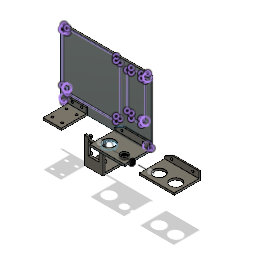
eye control mount (Autodesk Fusion 360 design; units mm, degrees)
Autodesk Fusion 360 part; units mm, degrees
sketch "Sketch1" plane through (0, 0, 0) normal (0, 0, 1) x (1, 0, 0)
  line L0 (-48.1387, 52.6701) -> (69.8353, 52.6701)
  line L1 (74.8353, 47.6701) -> (74.8353, -36.3099)
  line L2 (69.8353, -41.3099) -> (-48.1387, -41.3099)
  line L3 (-53.1387, -36.3099) -> (-53.1387, 47.6701)
  circle A0 centre (-46.9562, 49.6701) radius 1.5
  circle A1 centre (28.0438, 49.6701) radius 1.5
  circle A2 centre (-46.9562, -25.3299) radius 1.5
  circle A3 centre (28.0438, -25.3299) radius 1.5
  circle A4 centre (44.5655, 44.7298) radius 1
  circle A5 centre (63.5655, 44.7298) radius 1
  circle A6 centre (44.5655, -10.2702) radius 1
  circle A7 centre (63.5655, -10.2702) radius 1
  circle A8 centre (35.5562, -33.2226) radius 1.5
  circle A9 centre (65.5562, -33.2226) radius 1.5
  line L4 (25.4808, 51.0503) -> (25.4808, -28.2231)
  line L5 (-43.7955, -28.2231) -> (-43.7955, 51.0503)
  line L6 (41.0452, 42.402) -> (66.5755, 42.402)
  line L7 (66.5755, 42.402) -> (66.5755, -7.4237)
  line L8 (66.5755, -7.4237) -> (41.0452, -7.4237)
  line L9 (41.0452, -7.4237) -> (41.0452, 42.402)
  arc A10 (-48.1387, 52.6701) -> (-53.1387, 47.6701) centre (-48.1387, 47.6701) ccw
  arc A11 (74.8353, 47.6701) -> (69.8353, 52.6701) centre (69.8353, 47.6701) ccw
  arc A12 (69.8353, -41.3099) -> (74.8353, -36.3099) centre (69.8353, -36.3099) ccw
  arc A13 (-53.1387, -36.3099) -> (-48.1387, -41.3099) centre (-48.1387, -36.3099) ccw
  line L10 (46.8017, 47.9311) -> (61.294, 47.9311)
  line L11 (61.294, 47.9311) -> (61.294, -14.0499)
  line L12 (61.294, -14.0499) -> (46.8017, -14.0499)
  line L13 (46.8017, -14.0499) -> (46.8017, 47.9311)
  line L14 (-43.7955, -28.2231) -> (25.4808, -28.2231)
  line L15 (-43.7955, 51.0503) -> (25.4808, 51.0503)
  line L16 (-50.5532, 46.1259) -> (31.0875, 46.1259)
  line L17 (31.0875, 46.1259) -> (31.0875, -21.9998)
  line L18 (31.0875, -21.9998) -> (-50.5532, -21.9998)
  line L19 (-50.5532, -21.9998) -> (-50.5532, 46.1259)
  dimension "d1" = 3
  dimension "d4" = 75
  dimension "d5" = -75
  dimension "d6" = 2
  dimension "d9" = 19
  dimension "d10" = -55
  dimension "d11" = 3
  dimension "d14" = 30
  dimension "d15" = 0
  dimension "d30" = 5
  dimension "d31" = 5
  dimension "d59" = 8.0873
  dimension "d60" = 127.974
  dimension "d61" = 3
  dimension "d62" = 93.98
  dimension "d63" = 69.2762
  dimension "d65" = 75
  dimension "d66" = 75
  constraint horizontal L0
  constraint vertical L1
  constraint horizontal L2
  constraint vertical L3
  constraint vertical L4
  constraint vertical L5
  constraint horizontal L6
  constraint vertical L7
  constraint horizontal L8
  constraint vertical L9
  constraint tangent L0 A10
  constraint tangent L3 A10
  constraint tangent L0 A11
  constraint tangent L1 A11
  constraint tangent L1 A12
  constraint tangent L2 A12
  constraint equal A11 A12
  constraint tangent L2 A13
  constraint tangent L3 A13
  constraint equal A11 A13
  constraint horizontal L10
  constraint vertical L11
  constraint horizontal L12
  constraint vertical L13
  constraint horizontal L14
  constraint horizontal L15
  constraint horizontal L16
  constraint vertical L17
  constraint horizontal L18
  constraint vertical L19
  constraint coincident L5.end L15.start
  constraint coincident L4.start L15.end
  constraint coincident L5.start L14.start
  constraint coincident L4.end L14.end
  measures "d1" diameter of A0
  measures "d6" diameter of A4
  measures "d11" diameter of A8
  measures "d30" radius of A10
  measures "d31" radius of A11
  measures "d59" distance of L2 A8.centre
  measures "d60" distance of L1 L3
  measures "d61" distance of L0 A0.centre
  measures "d62" distance of L0 L2
  measures "d63" distance of L5.end L4.start
  measures "d65" distance of A0.centre A1.centre
  measures "d66" distance of A0.centre A2.centre
extrude "Extrude1" add sketch "Sketch1" along normal blind 2 makes body 1
sketch "Sketch2" plane through (0, 0, 0) normal (0, 0, -1) x (-1, 0, 0)
  circle A0 centre (46.9562, 49.6701) radius 1.5
  circle A1 centre (-28.0438, 49.6701) radius 1.5
  circle A2 centre (-63.5655, 44.7298) radius 1
  circle A3 centre (-28.0438, -25.3299) radius 1.5
  circle A4 centre (-44.5655, 44.7298) radius 1
  circle A5 centre (-65.5562, -33.2226) radius 1.5
  line L0 (43.7955, 51.0503) -> (43.7955, 46.1259)
  circle A6 centre (-44.5655, -10.2702) radius 1
  line L1 (-61.294, -7.4237) -> (-66.5755, -7.4237)
  line L2 (-66.5755, -7.4237) -> (-66.5755, 42.402)
  line L3 (-66.5755, 42.402) -> (-61.294, 42.402)
  line L4 (-41.0452, 42.402) -> (-41.0452, -7.4237)
  circle A7 centre (-63.5655, -10.2702) radius 1
  circle A8 centre (46.9562, -25.3299) radius 1.5
  circle A9 centre (-35.5562, -33.2226) radius 1.5
  line L5 (-69.8353, -41.3099) -> (48.1387, -41.3099)
  line L6 (53.1387, -36.3099) -> (53.1387, 47.6701)
  line L7 (48.1387, 52.6701) -> (-69.8353, 52.6701)
  line L8 (-74.8353, 47.6701) -> (-74.8353, -36.3099)
  arc A10 (53.1387, 47.6701) -> (48.1387, 52.6701) centre (48.1387, 47.6701) ccw
  arc A11 (-69.8353, 52.6701) -> (-74.8353, 47.6701) centre (-69.8353, 47.6701) ccw
  arc A12 (-74.8353, -36.3099) -> (-69.8353, -41.3099) centre (-69.8353, -36.3099) ccw
  arc A13 (48.1387, -41.3099) -> (53.1387, -36.3099) centre (48.1387, -36.3099) ccw
  line L9 (-61.294, 42.402) -> (-61.294, 47.9311)
  line L10 (-46.8017, 47.9311) -> (-46.8017, 42.402)
  line L11 (-46.8017, 42.402) -> (-41.0452, 42.402)
  line L12 (-25.4808, -21.9998) -> (-31.0875, -21.9998)
  line L13 (-31.0875, -21.9998) -> (-31.0875, 46.1259)
  line L14 (-31.0875, 46.1259) -> (-25.4808, 46.1259)
  line L15 (43.7955, -28.2231) -> (-25.4808, -28.2231)
  line L16 (-25.4808, -28.2231) -> (-25.4808, -21.9998)
  line L17 (-25.4808, 46.1259) -> (-25.4808, 51.0503)
  line L18 (-25.4808, 51.0503) -> (43.7955, 51.0503)
  line L19 (43.7955, 46.1259) -> (50.5532, 46.1259)
  line L20 (50.5532, 46.1259) -> (50.5532, -21.9998)
  line L21 (50.5532, -21.9998) -> (43.7955, -21.9998)
  line L22 (43.7955, -21.9998) -> (43.7955, -28.2231)
  line L23 (-41.0452, -7.4237) -> (-46.8017, -7.4237)
  line L24 (-46.8017, -14.0499) -> (-61.294, -14.0499)
  line L25 (-61.294, -14.0499) -> (-61.294, -7.4237)
  line L26 (-61.294, 47.9311) -> (-46.8017, 47.9311)
  line L27 (-46.8017, -7.4237) -> (-46.8017, -14.0499)
extrude "Extrude2" add sketch "Sketch2" along normal blind 0.6 contours L0 L12 L13 L14 L15 L16 L17 L18 L19 L20 L21 L22 | L1 L2 L3 L4 L9 L10 L11 L23 L24 L25 L26 L27 | L5 L6 L7 L8 A10 A11 A12 A13 bodies 1
sketch "Sketch1 (2)" plane through (0, 0, 2) normal (0, 0, 1) x (1, 0, 0) in component "switch mount"
  circle A0 centre (65.5562, -33.2226) radius 1.5
  circle A1 centre (63.5655, 44.7298) radius 1
  circle A2 centre (-46.9562, 49.6701) radius 1.5
  circle A3 centre (28.0438, 49.6701) radius 1.5
  circle A4 centre (-46.9562, -25.3299) radius 1.5
  circle A5 centre (44.5655, 44.7298) radius 1
  circle A6 centre (44.5655, -10.2702) radius 1
  circle A7 centre (63.5655, -10.2702) radius 1
  circle A8 centre (35.5562, -33.2226) radius 1.5
  circle A9 centre (28.0438, -25.3299) radius 1.5
  line L0 (-48.1387, -41.3099) -> (69.8353, -41.3099)
  line L1 (74.8353, -36.3099) -> (74.8353, 47.6701)
  line L2 (69.8353, 52.6701) -> (-48.1387, 52.6701)
  line L3 (-53.1387, 47.6701) -> (-53.1387, -36.3099)
  line L4 (36.9358, -28.4317) -> (74.2813, -28.4317)
  line L5 (74.2813, -28.4317) -> (74.2813, -40.7433)
  line L6 (74.2813, -40.7433) -> (25.2813, -40.7433)
  line L7 (25.2813, -40.7433) -> (25.2813, -34.7351)
  line L8 (-43.7955, -28.2231) -> (-43.7955, -21.9998)
  line L9 (66.5755, -7.4237) -> (61.294, -7.4237)
  line L10 (41.0452, -7.4237) -> (41.0452, 42.402)
  line L11 (41.0452, 42.402) -> (46.8017, 42.402)
  line L12 (66.5755, 42.402) -> (66.5755, -7.4237)
  arc A10 (-48.1387, 52.6701) -> (-53.1387, 47.6701) centre (-48.1387, 47.6701) ccw
  arc A11 (-53.1387, -36.3099) -> (-48.1387, -41.3099) centre (-48.1387, -36.3099) ccw
  arc A12 (69.8353, -41.3099) -> (74.8353, -36.3099) centre (69.8353, -36.3099) ccw
  arc A13 (74.8353, 47.6701) -> (69.8353, 52.6701) centre (69.8353, 47.6701) ccw
  line L13 (46.8017, -14.0499) -> (46.8017, -7.4237)
  line L14 (61.294, 47.9311) -> (61.294, 42.402)
  line L15 (61.294, 42.402) -> (66.5755, 42.402)
  line L16 (-50.5532, 46.1259) -> (-43.7955, 46.1259)
  line L17 (31.0875, 46.1259) -> (31.0875, -21.9998)
  line L18 (-43.7955, -21.9998) -> (-50.5532, -21.9998)
  line L19 (25.4808, -28.2231) -> (-43.7955, -28.2231)
  line L20 (-50.5532, -21.9998) -> (-50.5532, 46.1259)
  line L21 (-43.7955, 46.1259) -> (-43.7955, 51.0503)
  line L22 (-43.7955, 51.0503) -> (25.4808, 51.0503)
  line L23 (25.4808, 51.0503) -> (25.4808, 46.1259)
  line L24 (25.4808, -21.9998) -> (25.4808, -28.2231)
  line L25 (46.8017, -7.4237) -> (41.0452, -7.4237)
  line L26 (61.294, -14.0499) -> (46.8017, -14.0499)
  line L27 (46.8017, 47.9311) -> (61.294, 47.9311)
  line L28 (61.294, -7.4237) -> (61.294, -14.0499)
  line L29 (36.9358, -28.4317) -> (25.2813, -34.7351)
  line L30 (46.8017, 42.402) -> (46.8017, 47.9311)
  line L31 (25.4808, 46.1259) -> (31.0875, 46.1259)
  line L32 (31.0875, -21.9998) -> (25.4808, -21.9998)
  dimension "d55" = 49
  dimension "d56" = 12.3116
  dimension "d57" = 10.2749
  dimension "d58" = 4.7908
  constraint horizontal L4
  constraint vertical L5
  constraint horizontal L6
  constraint vertical L7
  measures "d55" distance of L5 L7
  measures "d56" distance of L4 L6
  measures "d57" distance of A8.centre L7
  measures "d58" distance of A8.centre L4
extrude "Extrude1'" add sketch "Sketch1 (2)" along normal blind 2 separate body contours L5 L6 A12 | L4 L5 L6 L7 A12 L29 makes body 2 in component "switch mount"
sketch "Sketch2 (2)" plane through (0, 0, 4) normal (0, 0, 1) x (1, 0, 0) in component "switch mount"
  circle A0 centre (65.5562, -33.2226) radius 1.5
  circle A1 centre (35.5562, -33.2226) radius 1.5
  line L0 (25.2813, -40.7433) -> (74.2813, -40.7433)
  line L1 (74.2813, -40.7433) -> (74.2813, -28.4317)
  line L2 (74.2813, -28.4317) -> (36.9358, -28.4317)
  line L3 (25.2813, -34.7351) -> (25.2813, -40.7433)
  line L4 (25.2813, -37.7433) -> (74.2813, -37.7433)
  line L5 (36.9358, -28.4317) -> (25.2813, -34.7351)
  dimension "d20" = 3
  constraint coincident L3 L4.start
  constraint coincident L1 L4.end
  constraint perpendicular L1 L4
  measures "d20" distance of L0 L4
extrude "Extrude2'" add sketch "Sketch2 (2)" along normal blind 35 contours L0 L1 L3 L4 bodies 2 in component "switch mount"
sketch "Sketch3" plane through (0, -40.7433, 0) normal (0, -1, 0) x (1, 0, 0) in component "switch mount"
  line L0 (25.2813, 2) -> (74.2813, 2)
  line L1 (74.2813, 2) -> (74.2813, 39)
  line L2 (74.2813, 39) -> (25.2813, 39)
  line L3 (25.2813, 39) -> (25.2813, 2)
  circle A0 centre (61.9113, 27) radius 5
  circle A1 centre (37.2813, 23.82) radius 8
  line L4 (27.2813, 27) -> (98.2678, 27) construction
  line L5 (74.2813, 29) -> (72.2813, 29)
  line L6 (72.2813, 29) -> (72.2813, 25)
  line L7 (72.2813, 25) -> (74.2813, 25)
  line L8 (74.2813, 25) -> (74.2813, 29)
  dimension "d23" = 10
  dimension "d50" = 16
  dimension "d53" = 12
  dimension "d81" = 12
  dimension "d82" = 12.37
  dimension "d83" = 2
  dimension "d84" = 2
  dimension "d85" = 2
  constraint coincident A0.centre L4
  constraint horizontal L5
  constraint vertical L6
  constraint horizontal L7
  constraint vertical L8
  constraint coincident L1 L5.start
  measures "d23" diameter of A0
  measures "d50" diameter of A1
  measures "d53" distance of L2 A0.centre
  measures "d81" distance of L3 A1.centre
  measures "d82" distance of L1 A0.centre
  measures "d83" distance of L6 L8
  measures "d84" distance of L4 L5
  measures "d85" distance of L4 L7
extrude "Extrude1''" add 1 faces at (74.2813, -39.7433, 15) along direction (1, 0, 0) blind 26 separate body on bodies 2 makes body 3 in component "eye power mount"
sketch "Sketch2 (3)" plane through (0, -40.7433, 0) normal (0, -1, 0) x (1, 0, 0) in component "eye power mount"
  line L0 (74.2813, 39) -> (74.2813, 2)
  line L1 (74.2813, 2) -> (100.2813, 2)
  line L2 (100.2813, 2) -> (100.2813, 39)
  line L3 (100.2813, 39) -> (74.2813, 39)
  circle A0 centre (80.2639, 31.6259) radius 1.5
  circle A1 centre (94.2639, 31.6259) radius 1.5
  circle A2 centre (80.2639, 11.6259) radius 1.5
  circle A3 centre (94.2639, 11.6259) radius 1.5
  dimension "d34" = 3
  dimension "d37" = 14
  dimension "d38" = -20
  dimension "d69" = 7.3741
  dimension "d70" = 5.9827
  measures "d34" diameter of A0
  measures "d69" distance of L3 A0.centre
  measures "d70" distance of L0 A0.centre
extrude "Extrude2''" cut sketch "Sketch2 (3)" against normal up to surface (3 mm away) contours A0 | A1 | A2 | A3 bodies 3 in component "eye power mount"
sketch "Sketch3 (2)" plane through (0, 0, 4) normal (0, 0, 1) x (1, 0, 0) in component "eye power mount"
  line L0 (74.2813, -28.4317) -> (74.2813, -37.7433)
  line L1 (74.2813, -37.7433) -> (100.2813, -37.7433)
  line L2 (100.2813, -37.7433) -> (100.2813, -28.4317)
  line L3 (100.2813, -28.4317) -> (74.2813, -28.4317)
  circle A0 centre (93.6757, -32.8867) radius 1.5
  circle A1 centre (80.6757, -32.8867) radius 1.5
  dimension "d41" = 3
  dimension "d44" = -13
  dimension "d45" = 0
  dimension "d71" = 4.455
  dimension "d72" = 6.6056
  measures "d41" diameter of A0
  measures "d71" distance of L3 A0.centre
  measures "d72" distance of L2 A0.centre
extrude "Extrude4" [suppressed]
extrude "Extrude4'" cut sketch "Sketch3 (2)" against normal up to surface (2 mm away) contours A0 | A1 bodies 3 in component "eye power mount"
extrude "Extrude5" cut sketch "Sketch3 (2)" against normal up to surface (4.6 mm away) contours A0 | A1 sketch seen with x (1, 0, 0) y (0, 1, 0) z (0, 0, 1) at (-115.1697, -0.5347, 0) bodies 1
sketch "Sketch4" plane through (0, 0, 4) normal (0, 0, 1) x (1, 0, 0) in component "eye power mount"
  circle A0 centre (80.6757, -32.8867) radius 1.5
  circle A1 centre (93.6757, -32.8867) radius 1.5
  line L0 (74.2813, -28.4317) -> (74.2813, -37.7433)
  line L1 (74.2813, -37.7433) -> (100.2813, -37.7433)
  line L2 (100.2813, -37.7433) -> (100.2813, -28.4317)
  line L3 (100.2813, -28.4317) -> (74.2813, -28.4317)
  line L4 (74.2813, -28.4317) -> (100.2813, -28.4317)
  line L5 (100.2813, -28.4317) -> (100.2813, -30.0261)
  line L6 (100.2813, -30.0261) -> (74.2813, -30.0261)
  line L7 (74.2813, -30.0261) -> (74.2813, -28.4317)
  constraint horizontal L4
  constraint vertical L5
  constraint horizontal L6
  constraint vertical L7
  constraint coincident L2 L5.end
  constraint coincident L0.start L3.end
extrude "Extrude5'" cut sketch "Sketch4" against normal up to surface (2 mm away) contours L0 L2 L3 L4 L5 L6 L7 bodies 3 in component "eye power mount"
sketch "Sketch1 (3)" plane through (0, 0, 2) normal (0, 0, 1) x (1, 0, 0) in component "TOF Sensor"
  line L0 (-16.31, -64.1211) -> (9.69, -64.1211)
  line L1 (9.69, -64.1211) -> (9.69, -101.6389)
  line L2 (9.69, -101.6389) -> (-16.31, -101.6389)
  line L3 (-16.31, -101.6389) -> (-16.31, -64.1211)
  circle A0 centre (-13.31, -67.1211) radius 1.5
  line L4 (1.4283, -74.6211) -> (1.4283, -79.6211) construction
  line L5 (-16.31, -98.6389) -> (9.69, -98.6389)
  circle A1 centre (6.69, -67.1211) radius 1.5
  circle A2 centre (-13.31, -87.1211) radius 1.5
  circle A3 centre (6.69, -87.1211) radius 1.5
  line L6 (-13.31, -67.1211) -> (-13.31, -87.1211) construction
  line L7 (-13.31, -87.1211) -> (6.69, -87.1211) construction
  line L8 (-13.31, -77.1211) -> (8.9688, -77.1211) construction
  line L9 (-3.31, -87.1211) -> (-3.31, -69.9219) construction
  line L10 (-8.31, -74.6211) -> (1.4521, -74.6211) construction
  line L11 (1.4521, -79.6211) -> (-8.31, -79.6211) construction
  line L12 (-8.31, -79.6211) -> (-8.31, -74.6211) construction
  line L13 (-11.11, -64.1211) -> (4.49, -64.1211)
  line L14 (4.49, -64.1211) -> (4.49, -67.4468)
  line L15 (4.49, -67.4468) -> (-11.11, -67.4468)
  line L16 (-11.11, -67.4468) -> (-11.11, -64.1211)
  circle A4 centre (-13.31, -67.1211) radius 2.5
  circle A5 centre (6.69, -67.1211) radius 2.5
  circle A6 centre (-13.31, -87.1211) radius 2.5
  circle A7 centre (6.69, -87.1211) radius 2.5
  line L17 (-10.81, -67.1211) -> (-10.81, -87.1211)
  line L18 (4.19, -67.1211) -> (4.19, -87.1211)
  line L19 (-10.81, -87.1211) -> (4.19, -87.1211)
  line L20 (-13.31, -69.6211) -> (6.69, -69.6211)
  point P0 (-13.31, -67.1211)
  dimension "d86" = 3
  dimension "d89" = 20
  dimension "d90" = -20
  dimension "d91" = 3
  dimension "d105" = 5
  dimension "d107" = 2.5
  dimension "d108" = 2.5
  dimension "d111" = 26
  dimension "d112" = 13
  dimension "d127" = 5
  dimension "d128" = 3.3257
  dimension "d129" = 34.5178
  dimension "d130" = 3
  dimension "d131" = 7.8
  dimension "d132" = 7.8
  constraint horizontal L0
  constraint vertical L1
  constraint horizontal L2
  constraint vertical L3
  constraint vertical L4
  constraint coincident L3 L5.start
  constraint coincident L1 L5.end
  constraint perpendicular L1 L5
  constraint coincident P0 A0.centre
  constraint coincident A2.centre L6.end
  constraint coincident A3.centre L7.end
  constraint midpoint L6 L8.start
  constraint midpoint L7 L9.start
  constraint horizontal L10
  constraint horizontal L11
  constraint vertical L12
  constraint vertical L9
  constraint horizontal L13
  constraint vertical L14
  constraint horizontal L15
  constraint vertical L16
  constraint coincident L0 L13.start
  constraint coincident L10 L4.start
  constraint coincident L11 L4.end
  constraint concentric A0 A4
  constraint perpendicular L8 L17
  constraint parallel L1 L18
  constraint tangent A4 L17
  constraint coincident A6 L17.end
  constraint coincident L7 L17.end
  constraint tangent A5 L18
  constraint coincident A7 L18.end
  constraint coincident L7 L18.end
  constraint coincident A4 L20.start
  constraint coincident L6 L20.start
  constraint coincident A5 L20.end
  constraint tangent A5 L20
  constraint coincident A4 L17.start
  constraint coincident A5 L18.start
  measures "d86" diameter of A0
  measures "d91" distance of L2 L5
  measures "d105" distance of L9 L12
  measures "d107" distance of L8 L11
  measures "d108" distance of L8 L10
  measures "d111" distance of L1 L3
  measures "d112" distance of L1 L9
  measures "d127" diameter of A4
  measures "d128" distance of L13 L15
  measures "d129" distance of L0 L5
  measures "d130" distance of L0 A1.centre
  measures "d131" distance of L9 L14
  measures "d132" distance of L9 L16
extrude "Extrude1'''" add sketch "Sketch1 (3)" along normal blind 3 separate body contours A7 | A6 | L0 L1 L3 L5 L14 L16 A4 A5 L17 L18 L19 L20 | L1 L2 L3 L5 | L15 L16 A4 | L14 L15 A5 | L15 A4 L17 L20 | L15 L17 L18 L20 | L15 A5 L18 L20 | A0 | A1 | A2 | A3 picked at (-11.349, -66.7594) picked at (4.7289, -66.7594) makes body 4 in component "TOF Sensor"
extrude "Extrude5''" add sketch "Sketch1 (3)" against normal blind 3 contours A7 | A6 | L15 L16 A4 | L14 L15 A5 picked at (-11.349, -66.7594) picked at (4.7289, -66.7594) bodies 4 in component "TOF Sensor"
extrude "Extrude3" add sketch "Sketch1 (3)" against normal blind 30 contours L1 L2 L3 L5 bodies 4 in component "TOF Sensor"
sketch "Sketch2 (4)" plane through (0, -98.6389, 0) normal (0, 1, 0) x (-1, 0, 0) in component "TOF Sensor"
  line L0 (16.31, -28) -> (16.31, 2)
  line L1 (-9.69, -28) -> (16.31, -28)
  line L2 (-9.69, 2) -> (-9.69, -28)
  circle A0 centre (12.2329, -20.7644) radius 1.5
  circle A1 centre (-4.5392, -20.7644) radius 1.5
  line L3 (16.31, -20.7644) -> (-9.69, -20.7644) construction
  line L4 (16.31, 2) -> (-9.69, 2)
  dimension "d98" = 3
  dimension "d99" = 3
  constraint coincident L0 L3.start
  constraint coincident L2 L3.end
  constraint perpendicular L2 L3
  constraint coincident A0.centre L3
  constraint coincident A1.centre L3
  measures "d98" diameter of A0
  measures "d99" diameter of A1
extrude "Extrude4''" cut sketch "Sketch2 (4)" against normal up to surface (3 mm away) contours A0 | A1 bodies 4 in component "TOF Sensor"
copy_body "CopyPasteBodies1" bodies 2 body 2 seen with x (1, 0, 0) y (0, 1, 0) z (0, 0, 1) at (-90, 0, 0) makes body 5 in component "mouth switch mount"
move_body "Move1" bodies 5 to x (1, 0, 0) y (0, 1, 0) z (0, 0, 1) at (70, 0, 0) in component "mouth switch mount"
extrude "Extrude5'''" cut sketch "Sketch3" against normal up to surface (3 mm away) contours L1 L5 L6 L7 L8 | A0 | A1 bodies 2 in component "switch mount"
sketch "Sketch1 (4)" plane through (0, -40.7433, 0) normal (0, -1, 0) x (1, 0, 0) in component "mouth switch mount"
  line L0 (5.2813, 2) -> (54.2813, 2)
  line L1 (54.2813, 2) -> (54.2813, 39)
  line L2 (54.2813, 39) -> (5.2813, 39)
  line L3 (5.2813, 39) -> (5.2813, 2)
  circle A0 centre (19.0928, 25.0845) radius 8
  circle A1 centre (42.453, 25.0845) radius 8
  line L4 (0.5125, 25.0845) -> (66.0078, 25.0845) construction
  dimension "d137" = 16
  dimension "d138" = 16
  constraint perpendicular L1 L4
  constraint coincident A0.centre L4
  constraint coincident A1.centre L4
  measures "d137" diameter of A0
  measures "d138" diameter of A1
extrude "Extrude1''''" cut sketch "Sketch1 (4)" against normal up to surface (3 mm away) contours A0 | A1 bodies 5 in component "mouth switch mount"
component "switch mount" placed x (1, 0, 0) y (0, 1, 0) z (0, 0, 1) at (0, 0, 0)
component "TOF Sensor" placed x (1, 0, 0) y (0, 1, 0) z (0, 0, 1) at (0, 0, 0)
component "eye power mount" placed x (1, 0, 0) y (0, 1, 0) z (0, 0, 1) at (-115.1697, -0.5347, 0)
component "eye switch mount" placed x (1, 0, 0) y (0, 1, 0) z (0, 0, 1) at (0, 0, 0) in component "switch mount"
component "mouth switch mount" placed x (1, 0, 0) y (0, 1, 0) z (0, 0, 1) at (90, 0, 0) in component "switch mount"
named bodies: "eye base plate"
